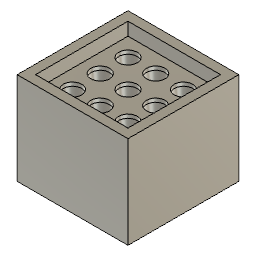
figitToy (Autodesk Fusion 360 design; units mm, degrees)
Autodesk Fusion 360 part; units mm, degrees
sketch "Sketch1" plane through (0, 0, 0) normal (0, 0, 1) x (1, 0, 0)
  line L0 (0, 0) -> (60, 0)
  line L1 (60, 0) -> (60, 60)
  line L2 (60, 60) -> (0, 60)
  line L3 (0, 60) -> (0, 0)
  line L4 (5, 5) -> (55, 5)
  line L5 (55, 5) -> (55, 55)
  line L6 (55, 55) -> (5, 55)
  line L7 (5, 55) -> (5, 5)
  dimension "d1" = 60
  dimension "d2" = 60
  constraint horizontal L0
  constraint vertical L1
  constraint horizontal L2
  constraint vertical L3
  constraint coincident L0.start L3.end
  constraint horizontal L4
  constraint vertical L5
  constraint horizontal L6
  constraint vertical L7
  measures "d1" distance of L0.start L0.end
  measures "d2" distance of L0.start L2.end
extrude "Extrude1" add sketch "Sketch1" along normal blind 50
extrude "Extrude2" add sketch "Sketch1" along normal blind 43 contours L4 L5 L6 L7
sketch "Sketch2" plane through (0, 0, 43) normal (0, 0, 1) x (-1, 0, 0)
  line L0 (-5, -55) -> (-5, -5)
  line L1 (-5, -5) -> (-55, -5)
  line L2 (-55, -5) -> (-55, -55)
  line L3 (-55, -55) -> (-5, -55)
  circle A0 centre (-15, -45) radius 5
  circle A1 centre (-30, -45) radius 5
  circle A2 centre (-45, -45) radius 5
  circle A3 centre (-15, -30) radius 5
  circle A4 centre (-30, -30) radius 5
  circle A5 centre (-45, -30) radius 5
  circle A6 centre (-15, -15) radius 5
  circle A7 centre (-30, -15) radius 5
  circle A8 centre (-45, -15) radius 5
  dimension "d7" = 10
  dimension "d8" = 10
  dimension "d9" = 10
  dimension "d10" = 10
  dimension "d11" = 10
  dimension "d12" = 10
  dimension "d13" = 10
  dimension "d14" = 10
  dimension "d15" = 10
  measures "d7" diameter of A0
  measures "d8" diameter of A1
  measures "d9" diameter of A2
  measures "d10" diameter of A3
  measures "d11" diameter of A4
  measures "d12" diameter of A5
  measures "d13" diameter of A6
  measures "d14" diameter of A7
  measures "d15" diameter of A8
hole "Hole1" at (45, 45, 43) at (45, 30, 43) at (45, 15, 43) at (30, 15, 43) at (30, 30, 43) at (30, 45, 43) at (15, 45, 43) at (15, 30, 43) at (15, 15, 43) direction (0, 0, -1) diameter 10 depth 2 tip angle 15
